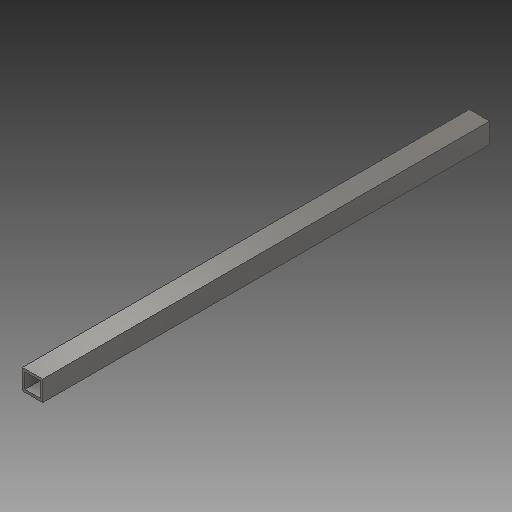
# Autodesk Inventor part: 22inSqTube
Saved by Autodesk Inventor 2018 (Build 220112000, 112)
## iProperties
Created: 2018-07-30
Part Number: 22inSqTube
Material: Steel, Mild
Document SubType Name: Modeling
Designer: Cole Tucker
Density: 7.85 g/cm^3
Appearance: Semi-Polished
Mass: 1238.15 g
Surface Area: 999.192 cm^2
Volume: 157.725 cm^3
Author: Cole Tucker
Autodesk Inventor part; units mm, degrees
ref_plane "YZ Plane" through (0, 0, 0) normal (1, 0, 0) x (0, 1, 0)
ref_plane "XZ Plane" through (0, 0, 0) normal (0, 1, 0) x (-1, 0, 0)
ref_plane "XY Plane" through (0, 0, 0) normal (0, 0, 1) x (1, 0, 0)
sketch "Sketch1" plane through (0, 0, 0) normal (0, 0, 1) x (1, 0, 0)
  line L0 (0, 0) -> (25.4, 0)
  line L1 (25.4, 0) -> (25.4, 25.4)
  line L2 (25.4, 25.4) -> (0, 25.4)
  line L3 (0, 25.4) -> (0, 0)
  line L4 (0, 0) -> (3.175, 0)
  line L5 (3.175, 0) -> (3.175, 3.175)
  line L6 (3.175, 3.175) -> (0, 3.175)
  line L7 (0, 3.175) -> (0, 0)
  line L8 (25.4, 25.4) -> (22.225, 25.4)
  line L9 (22.225, 25.4) -> (22.225, 22.225)
  line L10 (22.225, 22.225) -> (25.4, 22.225)
  line L11 (25.4, 22.225) -> (25.4, 25.4)
  line L12 (22.225, 22.225) -> (3.175, 22.225)
  line L13 (3.175, 22.225) -> (3.175, 3.175)
  line L14 (3.175, 3.175) -> (22.225, 3.175)
  line L15 (22.225, 3.175) -> (22.225, 22.225)
  dimension "d0" = 25.4
  dimension "d1" = 25.4
  dimension "d2" = 3.175
  dimension "d3" = 3.175
  dimension "d4" = 3.175
  dimension "d5" = 3.175
  constraints: 32 end point, 8 parallel, 4 horizontal, 4 perpendicular
  measures "d0" distance of L2.end L1.end
  measures "d1" distance of L1.end L0.end
  measures "d2" distance of L6.end L5.end
  measures "d3" distance of L5.end L4.end
  measures "d4" distance of L10.end L9.end
  measures "d5" distance of L9.end L8.end
extrude "Extrusion1" add sketch "Sketch1" along normal blind 558.8 contours L3 L6 L5 L0 | L5 L14 L15 L10 L1 L0 | L3 L2 L9 L12 L13 L6 | L10 L9 L2 L1
body "Solid1"
